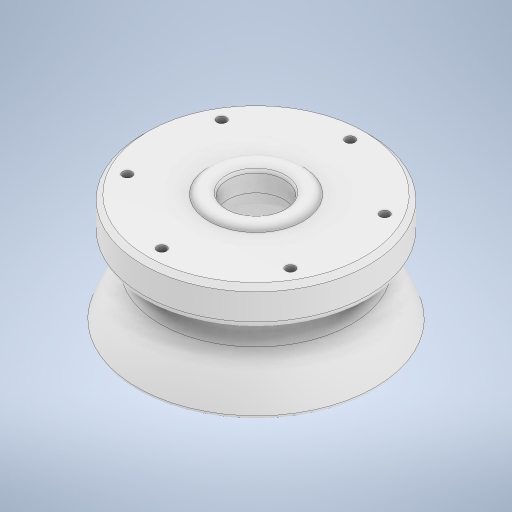
# Autodesk Inventor part: Bottom
Saved by Autodesk Inventor 2023 (Build 270158030, 158C)
## iProperties
Created: 2022-09-15
Part Number: Bottom
Material: ABS Plastic
Document SubType Name: Modeling
Designer: cjj5381
Density: 1.06 g/cm^3
Appearance: Smooth - White
Author: cjj5381
Autodesk Inventor part; units mm, degrees
ref_plane "YZ Plane" through (0, 0, 0) normal (1, 0, 0) x (0, 1, 0)
ref_plane "XZ Plane" through (0, 0, 0) normal (0, 1, 0) x (-1, 0, 0)
ref_plane "XY Plane" through (0, 0, 0) normal (0, 0, 1) x (1, 0, 0)
sketch "Sketch1" plane through (0, 0, 0) normal (0, 1, 0) x (-1, 0, 0)
  circle A0 centre (0, 0) radius 76.2
  dimension "d0" = 152.4
  constraints: 1 centre point, 1 coincident
  measures "d0" diameter of A0
extrude "Main-Body" add sketch "Sketch1" along normal blind 25.4
sketch "Sketch3" plane through (0, 0, 0) normal (0, 0, 1) x (1, 0, 0)
  line L0 (0, 25.4) -> (19.05, 25.4)
  line L1 (19.05, 25.4) -> (19.05, 12.7)
  line L2 (76.2, 25.4) -> (-76.2, 25.4) projected
  arc A0 (19.05, 12.7) -> (31.75, 0) centre (31.75, 12.7) ccw
  line L3 (76.2, 0) -> (-76.2, 0) projected
  line L4 (31.75, 0) -> (0, 0)
  line L5 (0, 0) -> (0, 25.4)
  dimension "d12" = 25.4
  dimension "d19" = 19.05
  constraints: 8 end point, 3 tangent, 2 collinear, 2 point on circle, 2 vertical, 1 centre point, 1 horizontal, 1 point on line
  measures "d12" diameter of A0
  measures "d19" distance of L0.start L0.end
revolve "Middle-Cutout" cut sketch "Sketch3" angle 360 about axis through (0, 0, 0) along (0, 1, 0)
sketch "Sketch4" plane through (0, 0, 0) normal (0, 0, 1) x (1, 0, 0)
  line L0 (76.2, 25.4) -> (-76.2, 25.4) projected
  line L1 (19.05, 25.4) -> (19.05, 12.7) projected
  arc A0 (31.75, 25.4) -> (19.05, 25.4) centre (25.4, 21.1879) ccw
  line L2 (31.75, 25.4) -> (19.05, 25.4)
  line L3 (0, 0) -> (0, 33.6646)
  dimension "d15" = 7.62
  dimension "d16" = 12.7
  constraints: 4 end point, 2 point on circle, 1 centre point, 1 collinear, 1 perpendicular, 1 point on line
  measures "d15" radius of A0
  measures "d16" distance of L1.start L2.start
revolve "Bump" add sketch "Sketch4" angle 360 about axis through (0, 0, 0) along (0, 1, 0)
fillet "Fillet1" radius 3.175 1 edges at (-19.05, 25.4, 0)
sketch "Sketch5" plane through (0, 0, 0) normal (0, 0, 1) x (1, 0, 0)
  line L0 (0, -64.4248) -> (0, 57.9021)
  arc A0 (74.5412, -50.5955) -> (27.2782, 0.8133) centre (0, -71.6953) ccw
  arc A1 (19.05, 12.7) -> (31.75, 0) centre (31.75, 12.7) ccw projected
  arc A2 (80.6512, -48.866) -> (43.4232, 0) centre (0, -71.6953) ccw
  line L1 (76.2, 0) -> (-76.2, 0) projected
  line L2 (43.4232, 0) -> (31.75, 0)
  arc A3 (19.05, 12.7) -> (31.75, 0) centre (31.75, 12.7) ccw projected
  arc A4 (27.2782, 0.8133) -> (31.75, 0) centre (31.75, 12.7) ccw
  line L3 (0, -71.6953) -> (80.6512, -48.866) construction
  line L4 (74.5412, -50.5955) -> (80.6512, -48.866)
  point P0 (0, 0)
  point P1 (27.2782, 0.8133)
  dimension "d29" = 154.94
  dimension "d30" = 6.35
  constraints: 8 end point, 7 point on circle, 4 point on line, 3 centre point, 2 collinear, 2 tangent, 1 vertical
  measures "d29" diameter of A0
  measures "d30" radial gap between concentric circles of A0 A2
revolve "Dome-Support" add sketch "Sketch5" angle 360 about axis through (0, -64.4248, 0) along (0, 1, 0)
fillet "Fillet2" radius 11.1125 1 edges at (-43.4232, 0, 0)
fillet "Fillet3" radius 1.5875 2 edges at (-74.5412, -50.5955, 0) (-80.6512, -48.866, 0)
fillet "Fillet4" radius 4.7625 1 edges at (76.2, 0, 0)
sketch "Sketch6" plane through (0, 25.4, 0) normal (0, 1, 0) x (1, 0, 0)
  line L0 (0, 0) -> (0, -63.5)
  point P0 (0, -63.5)
  dimension "d41" = 63.5
  constraints: 2 end point, 1 coincident, 1 vertical
  measures "d41" distance of L0.start L0.end
hole "Hole1" at (0, 25.4, 63.5) direction (0, -1, 0) diameter 6.4 depth 10.6
pattern_circular "Circular Pattern1" count 6 over 360 about axis through (0, 19.05, 0) along (0, -1, 0) of "Hole1"
chamfer "Chamfer1" distance 3.175 angle 45 1 edges at (76.2, 25.4, 0)
body "Solid1"
